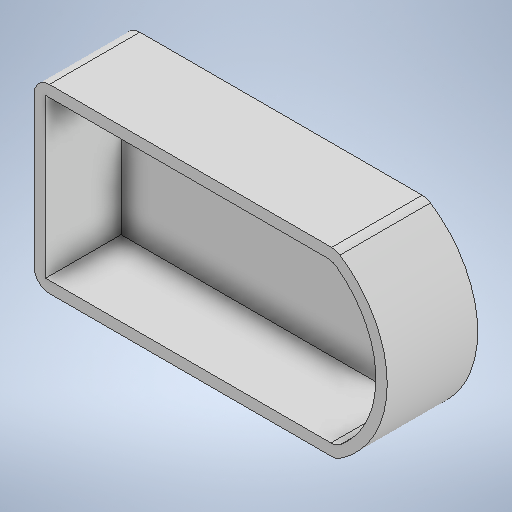
# Autodesk Inventor part: Couv
Saved by Autodesk Inventor 2025 (Build 290162000, 162)
## iProperties
Created: 2024-05-16
Part Number: Couv
Material: Générique
Document SubType Name: Modeling
Designer: luc4s
Density: 1 g/cm^3
Appearance: Par défaut
Author: luc4s
Autodesk Inventor part; units mm, degrees
ref_plane "YZ Plane" through (0, 0, 0) normal (1, 0, 0) x (0, 1, 0)
ref_plane "XZ Plane" through (0, 0, 0) normal (0, 1, 0) x (-1, 0, 0)
ref_plane "XY Plane" through (0, 0, 0) normal (0, 0, 1) x (1, 0, 0)
sketch "Esquisse1" plane through (0, 0, 0) normal (0, 0, 1) x (1, 0, 0)
  line L0 (0, 12) -> (-40, 12)
  line L1 (-40, 12) -> (-40, -12)
  line L2 (-40, -12) -> (0, -12)
  arc A0 (0, -12) -> (0, 12) centre (-7.2111, 0) ccw
  line L3 (-40, 0) -> (6.7889, 0) construction
  line L4 (-38.5, 10.5) -> (-0.5, 10.5)
  line L5 (0, -10.5) -> (-38.5, -10.5)
  line L6 (-38.5, -10.5) -> (-38.5, 10.5)
  line L7 (0, 14.6026) -> (0, -13.5331) construction
  arc A1 (0, -10.5) -> (-0.5, 10.5) centre (-7.4394, -0.1712) ccw
  point P0 (0, 0)
  point P1 (-19.5, 10.5)
  dimension "d0" = 40
  dimension "d1" = 24
  dimension "d2" = 1.5
  dimension "d3" = 1.5
  dimension "d4" = 1.5
  dimension "d6" = 14
  dimension "d8" = 38
  dimension "d9" = 12
  constraints: 16 end point, 5 point on circle, 3 point on line, 2 centre point, 2 horizontal, 2 midpoint, 2 parallel, 1 perpendicular, 1 vertical
  measures "d0" distance of L0.start L0.end
  measures "d1" distance of L0.end L1.end
  measures "d2" distance between parallel lines of L0 L4
  measures "d3" distance between parallel lines of L1 L6
  measures "d4" distance between parallel lines of L2 L5
  measures "d6" radius of A0
  measures "d8" distance of L4.start L4.end
  measures "d9" distance from line of L3 L0.end
extrude "Extrusion1" add sketch "Esquisse1" along normal blind 10
sketch "Esquisse2" plane through (0, 0, 0) normal (0, 0, -1) x (-1, 0, 0)
  arc A0 (0, 12) -> (0, -12) centre (7.2111, 0) ccw projected
  line L0 (40, -12) -> (0, -12) projected
  arc A1 (0, 12) -> (0, -12) centre (7.2111, 0) ccw
  line L1 (0, -12) -> (40, -12)
  line L2 (40, 12) -> (40, -12) projected
  line L3 (0, 12) -> (40, 12) projected
  line L4 (40, 12) -> (0, 12)
  point P0 (0, 0)
  constraints: 4 end point, 2 collinear, 2 point on circle, 1 centre point, 1 concentric
extrude "Extrusion2" add sketch "Esquisse2" along normal blind 2
fillet "Congé1" radius 2 2 edges at (-40, -12, 4) (-40, 12, 4)
fillet "Congé2" radius 2 2 edges at (0, 12, 4) (0, -12, 4)
fillet "Congé3" radius 2 2 edges at (-0.5, 10.5, 5) (0, -10.5, 5)
